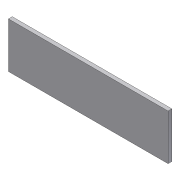
# Autodesk Inventor part: FE-00013-06
Saved by Autodesk Inventor 2012 (Build 160160000, 160)
## iProperties
Created: 2008-05-28
Part Number: FE-00013-06
Description: Bottom Plate
Document SubType Name: Modeling
Designer: narosenberg
Density: 1 g/cm^3
Mass: 129.048 g
Surface Area: 449.999 cm^2
Volume: 129.048 cm^3
Material: Default
Author: narosenberg
Autodesk Inventor part; units mm, degrees
ref_plane "YZ Plane" through (0, 0, 0) normal (1, 0, 0) x (0, 1, 0)
ref_plane "XZ Plane" through (0, 0, 0) normal (0, 1, 0) x (-1, 0, 0)
ref_plane "XY Plane" through (0, 0, 0) normal (0, 0, 1) x (1, 0, 0)
sketch "Sketch1" plane through (0, 0, 0) normal (0, 0, 1) x (1, 0, 0)
  line L0 (-264.0684, 73.4887) -> (2.6316, 73.4887)
  line L1 (2.6316, 73.4887) -> (2.6316, -2.7113)
  line L2 (2.6316, -2.7113) -> (-264.0684, -2.7113)
  line L3 (-264.0684, -2.7113) -> (-264.0684, 73.4887)
  dimension "d0" = 76.2
  dimension "d1" = 266.7
  constraints: 8 end point, 2 parallel, 1 horizontal, 1 perpendicular
  measures "d0" distance of L0.end L1.end
  measures "d1" distance of L1.end L2.end
extrude "Extrusion1" add sketch "Sketch1" along normal blind 6.35
body "Solid1"
